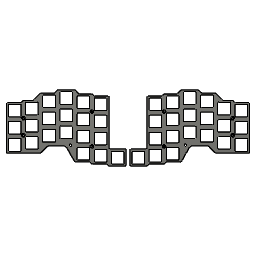
mriya-cnc-top-plate (Autodesk Fusion 360 design; units mm, degrees)
Autodesk Fusion 360 part; units mm, degrees
note: some values were not read from the file. Set by a fixed rule: which sketch regions a step uses.
sketch "mriya-top-plate" plane through (0, 0, 0) normal (0, 0, 1) x (1, 0, 0)
  line L0 (-96.0213, 15.6719) -> (-89.7787, 21.9145)
  line L1 (-21.4858, 1.079) -> (-22.6142, 2.2074)
  line L2 (-133.1, 14.7932) -> (-98.1426, 14.7932)
  line L3 (-39.0716, 2.7932) -> (-24.0284, 2.7932)
  line L4 (-3.6, 0.4932) -> (-20.0716, 0.4932)
  line L5 (-59.4741, 6.1094) -> (-67.7517, 20.7608)
  line L6 (-40.4858, 3.379) -> (-41.6142, 4.5074)
  line L7 (-117.6142, 71.579) -> (-116.4858, 72.7074)
  line L8 (-96.0716, 81.2932) -> (-82.2284, 81.2932)
  line L9 (-133.1, 70.9932) -> (-119.0284, 70.9932)
  line L10 (-87.6574, 22.7932) -> (-71.2344, 22.7932)
  line L11 (-43.0284, 5.0932) -> (-57.7328, 5.0932)
  line L12 (-77.0716, 84.7932) -> (-59.7284, 84.7932)
  line L13 (-53.5716, 80.2932) -> (-40.7284, 80.2932)
  line L14 (-19.9, 19.4932) -> (-2.9, 19.4932)
  line L15 (-20.9, 20.4932) -> (-20.9, 77.1932)
  line L16 (-78.4858, 84.2074) -> (-80.8142, 81.879)
  line L17 (-58.3142, 84.2074) -> (-54.9858, 80.879)
  line L18 (-134.6, 69.4932) -> (-134.6, 16.2932)
  line L19 (-38.1858, 78.579) -> (-39.3142, 79.7074)
  line L20 (-94.4, 40.3932) -> (-94.4, 27.9932)
  line L21 (-93.6, 41.1932) -> (-81.2, 41.1932)
  line L22 (-93.6, 27.1932) -> (-81.2, 27.1932)
  line L23 (-80.4, 40.3932) -> (-80.4, 27.9932)
  line L24 (-37.4, 56.0932) -> (-37.4, 43.6932)
  line L25 (-36.6, 56.8932) -> (-24.2, 56.8932)
  line L26 (-36.6, 42.8932) -> (-24.2, 42.8932)
  line L27 (-23.4, 56.0932) -> (-23.4, 43.6932)
  line L28 (-56.4, 58.3932) -> (-56.4, 45.9932)
  line L29 (-55.6, 59.1932) -> (-43.2, 59.1932)
  line L30 (-55.6, 45.1932) -> (-43.2, 45.1932)
  line L31 (-42.4, 58.3932) -> (-42.4, 45.9932)
  line L32 (-132.4, 68.0932) -> (-132.4, 55.6932)
  line L33 (-131.6, 68.8932) -> (-119.2, 68.8932)
  line L34 (-131.6, 54.8932) -> (-119.2, 54.8932)
  line L35 (-118.4, 68.0932) -> (-118.4, 55.6932)
  line L36 (-56.4, 39.3932) -> (-56.4, 26.9932)
  line L37 (-55.6, 40.1932) -> (-43.2, 40.1932)
  line L38 (-55.6, 26.1932) -> (-43.2, 26.1932)
  line L39 (-42.4, 39.3932) -> (-42.4, 26.9932)
  line L40 (-37.4, 18.0932) -> (-37.4, 5.6932)
  line L41 (-36.6, 18.8932) -> (-24.2, 18.8932)
  line L42 (-36.6, 4.8932) -> (-24.2, 4.8932)
  line L43 (-23.4, 18.0932) -> (-23.4, 5.6932)
  line L44 (-18.4, 15.7932) -> (-18.4, 3.3932)
  line L45 (-17.6, 16.5932) -> (-5.2, 16.5932)
  line L46 (-17.6, 2.5932) -> (-5.2, 2.5932)
  line L47 (-4.4, 15.7932) -> (-4.4, 3.3932)
  line L48 (-132.4, 49.0932) -> (-132.4, 36.6932)
  line L49 (-131.6, 49.8932) -> (-119.2, 49.8932)
  line L50 (-131.6, 35.8932) -> (-119.2, 35.8932)
  line L51 (-118.4, 49.0932) -> (-118.4, 36.6932)
  line L52 (-113.4, 51.3932) -> (-113.4, 38.9932)
  line L53 (-112.6, 52.1932) -> (-100.2, 52.1932)
  line L54 (-112.6, 38.1932) -> (-100.2, 38.1932)
  line L55 (-99.4, 51.3932) -> (-99.4, 38.9932)
  line L56 (-132.4, 30.0932) -> (-132.4, 17.6932)
  line L57 (-131.6, 30.8932) -> (-119.2, 30.8932)
  line L58 (-131.6, 16.8932) -> (-119.2, 16.8932)
  line L59 (-118.4, 30.0932) -> (-118.4, 17.6932)
  line L60 (-56.4, 20.3932) -> (-56.4, 7.9932)
  line L61 (-55.6, 21.1932) -> (-43.2, 21.1932)
  line L62 (-55.6, 7.1932) -> (-43.2, 7.1932)
  line L63 (-42.4, 20.3932) -> (-42.4, 7.9932)
  line L64 (-75.4, 43.8932) -> (-75.4, 31.4932)
  line L65 (-74.6, 44.6932) -> (-62.2, 44.6932)
  line L66 (-74.6, 30.6932) -> (-62.2, 30.6932)
  line L67 (-61.4, 43.8932) -> (-61.4, 31.4932)
  line L68 (-75.4, 81.8932) -> (-75.4, 69.4932)
  line L69 (-74.6, 82.6932) -> (-62.2, 82.6932)
  line L70 (-74.6, 68.6932) -> (-62.2, 68.6932)
  line L71 (-61.4, 81.8932) -> (-61.4, 69.4932)
  line L72 (-37.4, 37.0932) -> (-37.4, 24.6932)
  line L73 (-36.6, 37.8932) -> (-24.2, 37.8932)
  line L74 (-36.6, 23.8932) -> (-24.2, 23.8932)
  line L75 (-23.4, 37.0932) -> (-23.4, 24.6932)
  line L76 (-113.4, 32.3932) -> (-113.4, 19.9932)
  line L77 (-112.6, 33.1932) -> (-100.2, 33.1932)
  line L78 (-112.6, 19.1932) -> (-100.2, 19.1932)
  line L79 (-99.4, 32.3932) -> (-99.4, 19.9932)
  line L80 (-56.4, 77.3932) -> (-56.4, 64.9932)
  line L81 (-55.6, 78.1932) -> (-43.2, 78.1932)
  line L82 (-55.6, 64.1932) -> (-43.2, 64.1932)
  line L83 (-42.4, 77.3932) -> (-42.4, 64.9932)
  line L84 (-37.4, 75.0932) -> (-37.4, 62.6932)
  line L85 (-36.6, 75.8932) -> (-24.2, 75.8932)
  line L86 (-36.6, 61.8932) -> (-24.2, 61.8932)
  line L87 (-23.4, 75.0932) -> (-23.4, 62.6932)
  line L88 (-113.4, 70.3932) -> (-113.4, 57.9932)
  line L89 (-112.6, 71.1932) -> (-100.2, 71.1932)
  line L90 (-112.6, 57.1932) -> (-100.2, 57.1932)
  line L91 (-99.4, 70.3932) -> (-99.4, 57.9932)
  line L92 (-94.4, 59.3932) -> (-94.4, 46.9932)
  line L93 (-93.6, 60.1932) -> (-81.2, 60.1932)
  line L94 (-93.6, 46.1932) -> (-81.2, 46.1932)
  line L95 (-80.4, 59.3932) -> (-80.4, 46.9932)
  line L96 (-75.4, 62.8932) -> (-75.4, 50.4932)
  line L97 (-74.6, 63.6932) -> (-62.2, 63.6932)
  line L98 (-74.6, 49.6932) -> (-62.2, 49.6932)
  line L99 (-61.4, 62.8932) -> (-61.4, 50.4932)
  line L100 (-94.4, 78.3932) -> (-94.4, 65.9932)
  line L101 (-93.6, 79.1932) -> (-81.2, 79.1932)
  line L102 (-93.6, 65.1932) -> (-81.2, 65.1932)
  line L103 (-80.4, 78.3932) -> (-80.4, 65.9932)
  circle A0 centre (-115.9, 53.5432) radius 1
  circle A1 centre (-115.9, 34.5432) radius 1
  circle A2 centre (-63.5, 23.5932) radius 1.3
  circle A3 centre (-39.9, 22.5432) radius 1
  circle A4 centre (-39.9, 60.5432) radius 1
  arc A5 (-38.1858, 78.579) -> (-36.7716, 77.9932) centre (-36.7716, 79.9932) ccw
  arc A6 (-39.3142, 79.7074) -> (-40.7284, 80.2932) centre (-40.7284, 78.2932) ccw
  arc A7 (-54.9858, 80.879) -> (-53.5716, 80.2932) centre (-53.5716, 82.2931) ccw
  arc A8 (-58.3142, 84.2074) -> (-59.7284, 84.7932) centre (-59.7284, 82.7932) ccw
  arc A9 (-77.0716, 84.7932) -> (-78.4858, 84.2074) centre (-77.0716, 82.7933) ccw
  arc A10 (-82.2284, 81.2932) -> (-80.8142, 81.879) centre (-82.2284, 83.2932) ccw
  arc A11 (-96.0716, 81.2932) -> (-97.4858, 80.7074) centre (-96.0716, 79.2933) ccw
  arc A12 (-115.0716, 73.2932) -> (-116.4858, 72.7074) centre (-115.0716, 71.2933) ccw
  arc A13 (-119.0284, 70.9932) -> (-117.6142, 71.579) centre (-119.0284, 72.9932) ccw
  arc A14 (-133.1, 70.9932) -> (-134.6, 69.4932) centre (-133.1, 69.4932) ccw
  arc A15 (-134.6, 16.2932) -> (-133.1, 14.7932) centre (-133.1, 16.2932) ccw
  arc A16 (-98.1426, 14.7932) -> (-96.0213, 15.6719) centre (-98.1426, 17.7931) ccw
  arc A17 (-87.6574, 22.7932) -> (-89.7787, 21.9145) centre (-87.6573, 19.7931) ccw
  arc A18 (-67.7517, 20.7608) -> (-71.2344, 22.7932) centre (-71.2344, 18.793) ccw
  arc A19 (-59.4741, 6.1094) -> (-57.7328, 5.0932) centre (-57.7328, 7.0932) ccw
  arc A20 (-41.6142, 4.5074) -> (-43.0284, 5.0932) centre (-43.0284, 3.0933) ccw
  arc A21 (-40.4858, 3.379) -> (-39.0716, 2.7932) centre (-39.0716, 4.7932) ccw
  arc A22 (-22.6142, 2.2074) -> (-24.0284, 2.7932) centre (-24.0284, 0.7933) ccw
  arc A23 (-21.4858, 1.079) -> (-20.0716, 0.4932) centre (-20.0716, 2.4932) ccw
  arc A24 (-3.6, 0.4932) -> (-2.1, 1.9932) centre (-3.6, 1.9932) ccw
  line L104 (-2.1, 1.9932) -> (-2.1, 18.6932)
  line L105 (-36.7716, 77.9932) -> (-21.7, 77.9932)
  arc A25 (-131.6, 68.8932) -> (-132.4, 68.0932) centre (-131.6, 68.0932) ccw
  arc A26 (-118.4, 68.0932) -> (-119.2, 68.8932) centre (-119.2, 68.0932) ccw
  arc A27 (-119.2, 54.8932) -> (-118.4, 55.6932) centre (-119.2, 55.6932) ccw
  arc A28 (-132.4, 55.6932) -> (-131.6, 54.8932) centre (-131.6, 55.6932) ccw
  arc A29 (-131.6, 49.8932) -> (-132.4, 49.0932) centre (-131.6, 49.0932) ccw
  arc A30 (-118.4, 49.0932) -> (-119.2, 49.8932) centre (-119.2, 49.0932) ccw
  arc A31 (-119.2, 35.8932) -> (-118.4, 36.6932) centre (-119.2, 36.6932) ccw
  arc A32 (-132.4, 36.6932) -> (-131.6, 35.8932) centre (-131.6, 36.6932) ccw
  arc A33 (-131.6, 30.8932) -> (-132.4, 30.0932) centre (-131.6, 30.0932) ccw
  arc A34 (-118.4, 30.0932) -> (-119.2, 30.8932) centre (-119.2, 30.0932) ccw
  arc A35 (-119.2, 16.8932) -> (-118.4, 17.6932) centre (-119.2, 17.6932) ccw
  arc A36 (-132.4, 17.6932) -> (-131.6, 16.8932) centre (-131.6, 17.6932) ccw
  arc A37 (-113.4, 19.9932) -> (-112.6, 19.1932) centre (-112.6, 19.9932) ccw
  arc A38 (-100.2, 19.1932) -> (-99.4, 19.9932) centre (-100.2, 19.9932) ccw
  arc A39 (-99.4, 32.3932) -> (-100.2, 33.1932) centre (-100.2, 32.3932) ccw
  arc A40 (-112.6, 33.1932) -> (-113.4, 32.3932) centre (-112.6, 32.3932) ccw
  arc A41 (-100.2, 38.1932) -> (-99.4, 38.9932) centre (-100.2, 38.9932) ccw
  arc A42 (-113.4, 38.9932) -> (-112.6, 38.1932) centre (-112.6, 38.9932) ccw
  arc A43 (-112.6, 52.1932) -> (-113.4, 51.3932) centre (-112.6, 51.3932) ccw
  arc A44 (-99.4, 51.3932) -> (-100.2, 52.1932) centre (-100.2, 51.3932) ccw
  arc A45 (-113.4, 57.9932) -> (-112.6, 57.1932) centre (-112.6, 57.9932) ccw
  arc A46 (-100.2, 57.1932) -> (-99.4, 57.9932) centre (-100.2, 57.9932) ccw
  arc A47 (-99.4, 70.3932) -> (-100.2, 71.1932) centre (-100.2, 70.3932) ccw
  arc A48 (-112.6, 71.1932) -> (-113.4, 70.3932) centre (-112.6, 70.3932) ccw
  arc A49 (-93.6, 79.1932) -> (-94.4, 78.3932) centre (-93.6, 78.3932) ccw
  arc A50 (-80.4, 78.3932) -> (-81.2, 79.1932) centre (-81.2, 78.3932) ccw
  arc A51 (-81.2, 65.1932) -> (-80.4, 65.9932) centre (-81.2, 65.9932) ccw
  arc A52 (-94.4, 65.9932) -> (-93.6, 65.1932) centre (-93.6, 65.9932) ccw
  arc A53 (-93.6, 60.1932) -> (-94.4, 59.3932) centre (-93.6, 59.3932) ccw
  arc A54 (-80.4, 59.3932) -> (-81.2, 60.1932) centre (-81.2, 59.3932) ccw
  arc A55 (-81.2, 46.1932) -> (-80.4, 46.9932) centre (-81.2, 46.9932) ccw
  arc A56 (-94.4, 46.9932) -> (-93.6, 46.1932) centre (-93.6, 46.9932) ccw
  arc A57 (-93.6, 41.1932) -> (-94.4, 40.3932) centre (-93.6, 40.3932) ccw
  arc A58 (-94.4, 27.9932) -> (-93.6, 27.1932) centre (-93.6, 27.9932) ccw
  arc A59 (-81.2, 27.1932) -> (-80.4, 27.9932) centre (-81.2, 27.9932) ccw
  arc A60 (-80.4, 40.3932) -> (-81.2, 41.1932) centre (-81.2, 40.3932) ccw
  arc A61 (-75.4, 31.4932) -> (-74.6, 30.6932) centre (-74.6, 31.4932) ccw
  arc A62 (-74.6, 44.6932) -> (-75.4, 43.8932) centre (-74.6, 43.8932) ccw
  arc A63 (-61.4, 43.8932) -> (-62.2, 44.6932) centre (-62.2, 43.8932) ccw
  arc A64 (-62.2, 30.6932) -> (-61.4, 31.4932) centre (-62.2, 31.4932) ccw
  arc A65 (-62.2, 49.6932) -> (-61.4, 50.4932) centre (-62.2, 50.4932) ccw
  arc A66 (-75.4, 50.4932) -> (-74.6, 49.6932) centre (-74.6, 50.4932) ccw
  arc A67 (-74.6, 63.6932) -> (-75.4, 62.8932) centre (-74.6, 62.8932) ccw
  arc A68 (-61.4, 62.8932) -> (-62.2, 63.6932) centre (-62.2, 62.8932) ccw
  arc A69 (-62.2, 68.6932) -> (-61.4, 69.4932) centre (-62.2, 69.4932) ccw
  arc A70 (-75.4, 69.4932) -> (-74.6, 68.6932) centre (-74.6, 69.4932) ccw
  arc A71 (-74.6, 82.6932) -> (-75.4, 81.8932) centre (-74.6, 81.8932) ccw
  arc A72 (-61.4, 81.8932) -> (-62.2, 82.6932) centre (-62.2, 81.8932) ccw
  arc A73 (-55.6, 78.1932) -> (-56.4, 77.3932) centre (-55.6, 77.3932) ccw
  arc A74 (-56.4, 64.9932) -> (-55.6, 64.1932) centre (-55.6, 64.9932) ccw
  arc A75 (-43.2, 64.1932) -> (-42.4, 64.9932) centre (-43.2, 64.9932) ccw
  arc A76 (-42.4, 77.3932) -> (-43.2, 78.1932) centre (-43.2, 77.3932) ccw
  arc A77 (-42.4, 58.3932) -> (-43.2, 59.1932) centre (-43.2, 58.3932) ccw
  arc A78 (-55.6, 59.1932) -> (-56.4, 58.3932) centre (-55.6, 58.3932) ccw
  arc A79 (-56.4, 45.9932) -> (-55.6, 45.1932) centre (-55.6, 45.9932) ccw
  arc A80 (-43.2, 45.1932) -> (-42.4, 45.9932) centre (-43.2, 45.9932) ccw
  arc A81 (-42.4, 39.3932) -> (-43.2, 40.1932) centre (-43.2, 39.3932) ccw
  arc A82 (-55.6, 40.1932) -> (-56.4, 39.3932) centre (-55.6, 39.3932) ccw
  arc A83 (-56.4, 26.9932) -> (-55.6, 26.1932) centre (-55.6, 26.9932) ccw
  arc A84 (-43.2, 26.1932) -> (-42.4, 26.9932) centre (-43.2, 26.9932) ccw
  arc A85 (-42.4, 20.3932) -> (-43.2, 21.1932) centre (-43.2, 20.3932) ccw
  arc A86 (-55.6, 21.1932) -> (-56.4, 20.3932) centre (-55.6, 20.3932) ccw
  arc A87 (-56.4, 7.9932) -> (-55.6, 7.1932) centre (-55.6, 7.9932) ccw
  arc A88 (-43.2, 7.1932) -> (-42.4, 7.9932) centre (-43.2, 7.9932) ccw
  arc A89 (-37.4, 5.6932) -> (-36.6, 4.8932) centre (-36.6, 5.6932) ccw
  arc A90 (-24.2, 4.8932) -> (-23.4, 5.6932) centre (-24.2, 5.6932) ccw
  arc A91 (-23.4, 18.0932) -> (-24.2, 18.8932) centre (-24.2, 18.0932) ccw
  arc A92 (-36.6, 18.8932) -> (-37.4, 18.0932) centre (-36.6, 18.0932) ccw
  arc A93 (-18.4, 3.3932) -> (-17.6, 2.5932) centre (-17.6, 3.3932) ccw
  arc A94 (-5.2, 2.5932) -> (-4.4, 3.3932) centre (-5.2, 3.3932) ccw
  arc A95 (-4.4, 15.7932) -> (-5.2, 16.5932) centre (-5.2, 15.7932) ccw
  arc A96 (-17.6, 16.5932) -> (-18.4, 15.7932) centre (-17.6, 15.7932) ccw
  arc A97 (-24.2, 23.8932) -> (-23.4, 24.6932) centre (-24.2, 24.6932) ccw
  arc A98 (-37.4, 24.6932) -> (-36.6, 23.8932) centre (-36.6, 24.6932) ccw
  arc A99 (-36.6, 37.8932) -> (-37.4, 37.0932) centre (-36.6, 37.0932) ccw
  arc A100 (-23.4, 37.0932) -> (-24.2, 37.8932) centre (-24.2, 37.0932) ccw
  arc A101 (-24.2, 42.8932) -> (-23.4, 43.6932) centre (-24.2, 43.6932) ccw
  arc A102 (-37.4, 43.6932) -> (-36.6, 42.8932) centre (-36.6, 43.6932) ccw
  arc A103 (-36.6, 56.8932) -> (-37.4, 56.0932) centre (-36.6, 56.0932) ccw
  arc A104 (-23.4, 56.0932) -> (-24.2, 56.8932) centre (-24.2, 56.0932) ccw
  arc A105 (-24.2, 61.8932) -> (-23.4, 62.6932) centre (-24.2, 62.6932) ccw
  arc A106 (-37.4, 62.6932) -> (-36.6, 61.8932) centre (-36.6, 62.6932) ccw
  arc A107 (-36.6, 75.8932) -> (-37.4, 75.0932) centre (-36.6, 75.0932) ccw
  arc A108 (-23.4, 75.0932) -> (-24.2, 75.8932) centre (-24.2, 75.0932) ccw
  arc A109 (-2.1, 18.6932) -> (-2.9, 19.4932) centre (-2.9, 18.6932) ccw
  arc A110 (-20.9, 77.1932) -> (-21.7, 77.9932) centre (-21.7, 77.1932) ccw
  circle A111 centre (-115.9, 53.5432) radius 2
  circle A112 centre (-115.9, 34.5432) radius 2
  circle A113 centre (-39.9, 22.5432) radius 2
  circle A114 centre (-39.9, 60.5432) radius 2
  line L106 (-104.0213, 74.1719) -> (-97.4858, 80.7074)
  line L107 (-106.1426, 73.2932) -> (-115.0716, 73.2932)
  arc A115 (-106.1426, 73.2932) -> (-104.0213, 74.1719) centre (-106.1426, 76.2932) ccw
  arc A116 (-20.9, 20.4932) -> (-19.9, 19.4932) centre (-19.9, 20.4932) ccw
  dimension "d1" = 2
  dimension "d2" = 2
  dimension "d3" = 2.6
  dimension "d4" = 2
  dimension "d5" = 2
  dimension "d17" = 4
  dimension "d18" = 4
  dimension "d19" = 4
  dimension "d20" = 4
  constraint tangent L19 A5
  constraint tangent L19 A6
  constraint tangent L13 A7
  constraint tangent L17 A8
  constraint tangent L12 A9
  constraint tangent L16 A10
  constraint tangent L8 A11
  constraint tangent L7 A13
  constraint tangent L9 A14
  constraint tangent L18 A15
  constraint tangent L2 A16
  constraint tangent L0 A17
  constraint tangent L10 A18
  constraint tangent L5 A19
  constraint tangent L11 A20
  constraint tangent L6 A21
  constraint tangent L3 A22
  constraint tangent L1 A23
  constraint tangent L4 A24
  constraint tangent A24 L104
  constraint perpendicular L104 L105
  constraint perpendicular L15 L105
  constraint perpendicular L14 L104
  constraint tangent L32 A25
  constraint tangent L33 A26
  constraint tangent L35 A27
  constraint tangent L34 A28
  constraint tangent L49 A29
  constraint tangent L49 A30
  constraint tangent L51 A31
  constraint tangent L50 A32
  constraint tangent L57 A33
  constraint tangent L57 A34
  constraint tangent L59 A35
  constraint tangent L58 A36
  constraint tangent L76 A37
  constraint tangent L78 A38
  constraint tangent L79 A39
  constraint tangent L77 A40
  constraint tangent L54 A41
  constraint tangent L54 A42
  constraint tangent L52 A43
  constraint tangent L53 A44
  constraint tangent L90 A45
  constraint tangent L90 A46
  constraint tangent L91 A46
  constraint tangent L91 A47
  constraint tangent L89 A48
  constraint tangent L100 A49
  constraint tangent L101 A50
  constraint tangent L103 A51
  constraint tangent L102 A52
  constraint tangent L93 A53
  constraint tangent L93 A54
  constraint tangent L95 A55
  constraint tangent L94 A56
  constraint tangent L21 A57
  constraint tangent L20 A58
  constraint tangent L22 A58
  constraint tangent L22 A59
  constraint tangent L23 A60
  constraint tangent L64 A61
  constraint tangent L66 A61
  constraint tangent L64 A62
  constraint tangent L65 A63
  constraint tangent L67 A64
  constraint tangent L98 A65
  constraint tangent L98 A66
  constraint tangent L96 A67
  constraint tangent L97 A68
  constraint tangent L70 A69
  constraint tangent L70 A70
  constraint tangent L68 A71
  constraint tangent L69 A72
  constraint tangent L80 A73
  constraint tangent L80 A74
  constraint tangent L82 A74
  constraint tangent L82 A75
  constraint tangent L83 A75
  constraint tangent L83 A76
  constraint tangent L81 A76
  constraint tangent L29 A77
  constraint tangent L29 A78
  constraint tangent L28 A79
  constraint tangent L30 A80
  constraint tangent L37 A81
  constraint tangent L37 A82
  constraint tangent L36 A82
  constraint tangent L36 A83
  constraint tangent L38 A83
  constraint tangent L38 A84
  constraint tangent L39 A84
  constraint tangent L61 A85
  constraint tangent L61 A86
  constraint tangent L60 A86
  constraint tangent L60 A87
  constraint tangent L62 A88
  constraint tangent L40 A89
  constraint tangent L42 A90
  constraint tangent L43 A91
  constraint tangent L41 A91
  constraint tangent L41 A92
  constraint tangent L40 A92
  constraint tangent L44 A93
  constraint tangent L46 A93
  constraint tangent L46 A94
  constraint tangent L47 A94
  constraint tangent L47 A95
  constraint tangent L45 A95
  constraint tangent L45 A96
  constraint tangent L44 A96
  constraint tangent L74 A97
  constraint tangent L75 A97
  constraint tangent L74 A98
  constraint tangent L72 A99
  constraint tangent L73 A100
  constraint tangent L26 A101
  constraint tangent L27 A101
  constraint tangent L26 A102
  constraint tangent L24 A103
  constraint tangent L25 A104
  constraint tangent L86 A105
  constraint tangent L87 A105
  constraint tangent L86 A106
  constraint tangent L84 A107
  constraint tangent L85 A108
  constraint tangent L104 A109
  constraint tangent L14 A109
  constraint tangent L15 A110
  constraint tangent L105 A110
  constraint concentric A0 A111
  constraint concentric A1 A112
  constraint concentric A3 A113
  constraint concentric A4 A114
  constraint tangent A11 L106
  constraint tangent A12 L107
  constraint tangent L106 A115
  constraint tangent L107 A115
  constraint horizontal L14
  constraint tangent L15 A116
  constraint tangent L14 A116
  measures "d1" diameter of A0
  measures "d2" diameter of A1
  measures "d3" diameter of A2
  measures "d4" diameter of A3
  measures "d5" diameter of A4
  measures "d17" diameter of A111
  measures "d18" diameter of A112
  measures "d19" diameter of A113
  measures "d20" diameter of A114
extrude "Extrude1" add sketch "mriya-top-plate" along normal blind 1.5 contours L0 L1 L2 L3 L4 L5 L6 L7 L8 L9 L10 L11 L12 L13 L14 L15 L16 L17 L18 L19 A5 A6 A7 A8 A9 A10 A11 A12 A13 A14 A15 A16 A17 A18 A19 A20 A21 A22 A23 A24 L104 L105 A109 A110 L106 L107 A115 A116 makes body 1
extrude "Extrude2" add sketch "mriya-top-plate" along normal blind 0.8 contours A111 | A112 | A113 | A114 bodies 1
mirror "Mirror1" about plane through (0, 0, 0) normal (1, 0, 0) of bodies 1 makes body 2
named bodies: "Left", "Right"
